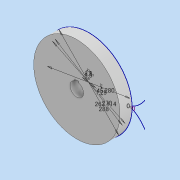
# Autodesk Inventor part: gear2
Saved by Autodesk Inventor 2022 (Build 260153000, 153)
## iProperties
Created: 2023-12-21
Part Number: gear2
Material: 一般
Document SubType Name: Modeling
Designer: ktamu
Density: 1 g/cm^3
Appearance: 既定
Author: ktamu
Autodesk Inventor part; units mm, degrees
ref_plane "YZ Plane" through (0, 0, 0) normal (1, 0, 0) x (0, 1, 0)
ref_plane "XZ Plane" through (0, 0, 0) normal (0, 1, 0) x (-1, 0, 0)
ref_plane "XY Plane" through (0, 0, 0) normal (0, 0, 1) x (1, 0, 0)
sketch "スケッチ1" plane through (0, 0, 0) normal (0, 0, 1) x (1, 0, 0)
  circle A0 centre (0, 0) radius 144
  arc A1 (-6.699441, 21.479467) -> (7, 21.383405) centre (0, 0) ccw
  line L0 (0, 22.5) -> (0, 17)
  line L1 (0, 22.5) -> (0, 26.3)
  line L2 (0, 26.3) -> (7, 26.3)
  line L3 (7, 26.3) -> (7, 21.383405)
  line L4 (7, 17) -> (0, 17)
  line L5 (-6.699441, 21.479467) -> (-6.699441, 26.3)
  line L6 (-6.699441, 26.3) -> (0, 26.3)
  circle A2 centre (0, 0) radius 135 construction
  circle A3 centre (0, 0) radius 131.55695 construction
  circle A4 centre (0, 0) radius 140 construction
  line L7 (0, 0) -> (139.964753, 3.141329)
  line L8 (0, 0) -> (140, 0) construction
  line L9 (0, 0) -> (134.981058, 2.261433)
  arc A5 (131.55695, 0) -> (131.538491, 2.203757) centre (0, 0) ccw
  line L10 (150.184159, 7.263201) -> (152.050707, -0.299145)
  line L11 (119.584335, 0) -> (125.15167, 0)
  circle A6 centre (0, 0) radius 131.55695 construction
  line L12 (0, 0) -> (134.981058, -2.261433)
  line L13 (150.184159, -7.263201) -> (152.050707, 0.299145)
  arc A7 (131.538491, -2.203757) -> (131.55695, 0) centre (0, 0) ccw
  line L14 (143.93152, 4.440455) -> (146.480822, 0.114106)
  line L15 (146.480822, 0.114106) -> (143.93152, -4.440455)
  line L16 (134.979291, 2.261403) -> (134.981058, 2.261433)
  line L17 (134.907008, -2.260192) -> (135.074128, -2.262992)
  line L18 (143.93152, -4.440455) -> (144.436873, -3.537595)
  line L19 (143.93152, 4.440455) -> (145.266584, 2.433754)
  line L20 (145.266584, 2.433754) -> (146.480822, 0.114106)
  line L21 (131.538491, 2.203757) -> (134.981058, 2.261433)
  line L22 (131.538491, -2.203757) -> (135.074128, -2.262992)
  line L23 (131.570586, -2.204295) -> (131.538491, -2.203757)
  arc A8 (131.538491, -2.203757) -> (131.538491, -2.203757) centre (131.538491, -2.203757) ccw
  line L24 (131.7018, 2.206493) -> (131.538491, 2.203757)
  dimension "d7" = 270
  dimension "d9" = 280
  dimension "d0" = 288
  dimension "d1" = 45
  dimension "d2" = 5.5
  dimension "d3" = 3.8
  dimension "d4" = 7
  dimension "d8" = 263.1139
  dimension "d18" = 1.28571
  dimension "d19" = 0
  constraints: 50 end point, 13 point on line, 12 point on circle, 7 coincident, 6 centre point, 4 collinear, 3 horizontal, 3 perpendicular, 3 symmetric about line, 2 coincident with centre, 2 tangent, 2 vertical, 1 equal length, 1 line through centre, 23 other
  measures "d0" diameter of A0
  measures "d1" diameter of A1
  measures "d2" distance of L0.end L0.start
  measures "d3" distance of L0.start L1.end
  measures "d4" distance of L1.end L2.end
  measures "d8" diameter of A3
  measures "d18" angle of L8 L7
  measures "d19" diameter of A8
sketch "スケッチ1 outline for 押し出し1" plane through (0, 0, 0) normal (0, 0, 1) x (1, 0, 0)
  circle A0 centre (0, 0) radius 144
  line L0 (0, 26.3) -> (7, 26.3)
  line L1 (-6.699441, 26.3) -> (0, 26.3)
  line L2 (-6.699441, 21.479467) -> (-6.699441, 26.3)
  arc A1 (7, 21.383405) -> (-6.699441, 21.479467) centre (0, 0) cw
  line L3 (7, 26.3) -> (7, 21.383405)
extrude "押し出し1" add sketch "スケッチ1 outline for 押し出し1" along normal blind 40
sketch "スケッチ2" plane through (0, 0, 0) normal (0, 0, -1) x (-1, 0, 0)
  point P0 (0, 0)
